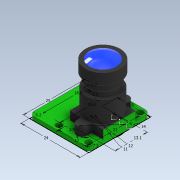
# Autodesk Inventor part: Arducam Camera
Saved by Autodesk Inventor 2020 (Build 240168000, 168)
## iProperties
Created: 2020-12-28
Part Number: Arducam Camera
Material: Generic
Document SubType Name: Modeling
Designer: DELL
Density: 1 g/cm^3
Appearance: Default
Author: DELL
Autodesk Inventor part; units mm, degrees
ref_plane "YZ Plane" through (0, 0, 0) normal (1, 0, 0) x (0, 1, 0)
ref_plane "XZ Plane" through (0, 0, 0) normal (0, 1, 0) x (-1, 0, 0)
ref_plane "XY Plane" through (0, 0, 0) normal (0, 0, 1) x (1, 0, 0)
sketch "Sketch1" plane through (0, 0, 0) normal (0, 1, 0) x (-1, 0, 0)
  line L0 (12, -12.5) -> (-12, -12.5)
  line L1 (-12, -12.5) -> (-12, 12.5)
  line L2 (-12, 12.5) -> (12, 12.5)
  line L3 (12, 12.5) -> (12, -12.5)
  line L4 (12, -12.5) -> (-12, 12.5) construction
  line L5 (-12, -12.5) -> (12, 12.5) construction
  circle A0 centre (2, 10.5) radius 1.25
  circle A1 centre (-10, 10.5) radius 1.25
  circle A2 centre (2, -10.5) radius 1.25
  circle A3 centre (-10, -10.5) radius 1.25
  line L6 (12, 0) -> (-12, 0) construction
  line L7 (10.1, -8.3) -> (11.8, -8.3)
  line L8 (11.8, -8.3) -> (11.8, 8.3)
  line L9 (11.8, 8.3) -> (10.1, 8.3)
  line L10 (10.1, 8.3) -> (10.1, -8.3)
  line L11 (10.1, -8.3) -> (11.8, 8.3) construction
  line L12 (11.8, -8.3) -> (10.1, 8.3) construction
  line L13 (6.6, -7.8) -> (10.1, -7.8)
  line L14 (10.1, -7.8) -> (10.1, 7.8)
  line L15 (10.1, 7.8) -> (6.6, 7.8)
  line L16 (6.6, 7.8) -> (6.6, -7.8)
  line L17 (6.6, -7.8) -> (10.1, 7.8) construction
  line L18 (10.1, -7.8) -> (6.6, 7.8) construction
  line L19 (1.5, -6.55) -> (-12, -6.55)
  line L20 (-12, -6.55) -> (-12, 6.55)
  line L21 (-12, 6.55) -> (1.5, 6.55)
  line L22 (1.5, 6.55) -> (1.5, -6.55)
  line L23 (1.5, -6.55) -> (-12, 6.55) construction
  line L24 (-12, -6.55) -> (1.5, 6.55) construction
  circle A4 centre (-5.25, 0) radius 6.75
  line L25 (-5.25, 6.55) -> (-5.25, -6.55) construction
  line L26 (-3.25, 8.55) -> (-3.25, -6.55)
  line L27 (-7.25, -8.55) -> (-7.25, 8.55)
  circle A5 centre (-5.25, 8.55) radius 2
  circle A6 centre (-5.25, -8.55) radius 2
  line L28 (-3.25, -8.55) -> (-3.25, -6.55)
  circle A7 centre (-5.25, 0) radius 6
  circle A8 centre (-5.25, 0) radius 5.5
  circle A9 centre (-5.25, 0) radius 7
  point P0 (0, 0)
  point P1 (10.95, 0)
  point P2 (8.35, 0)
  point P3 (-12, 1.854)
  point P4 (-12, -1.854)
  point P5 (-7.7193, -6.55)
  point P6 (-7.25, -6.7082)
  point P7 (-3.25, -6.7082)
  point P8 (-2.7807, -6.55)
  point P9 (-2.7807, 6.55)
  point P10 (-3.25, 6.7082)
  point P11 (-7.25, 6.7082)
  point P12 (-7.7193, 6.55)
  point P13 (12, -8.3)
  dimension "d0" = 25
  dimension "d1" = 24
  dimension "d2" = 2.5
  dimension "d3" = 21
  dimension "d4" = 12
  dimension "d5" = 2
  dimension "d6" = 16.6
  dimension "d7" = 1.7
  dimension "d8" = 15.6
  dimension "d9" = 3.5
  dimension "d10" = 13.5
  dimension "d11" = 13.1
  dimension "d12" = 4
  dimension "d13" = 4
  dimension "d14" = 11
  dimension "d15" = 12
  dimension "d16" = 14
  dimension "d35" = 0.2
  constraints: 58 end point, 12 midpoint, 9 centre point, 9 parallel, 6 point on line, 5 perpendicular, 4 coincident, 4 equal radius, 4 horizontal, 4 point on circle, 4 tangent, 3 horizontal alignment, 2 symmetric about line, 2 vertical alignment, 1 vertical, 3 other
  measures "d0" distance of L2.end L0.start
  measures "d1" distance of L1.end L2.end
  measures "d2" diameter of A0
  measures "d3" distance of A3.centre A1.centre
  measures "d4" distance of A1.centre A0.centre
  measures "d5" distance from line of L1 A1.centre
  measures "d6" distance between parallel lines of L7 L9
  measures "d7" distance of L7.start L7.end
  measures "d8" distance of L15.end L13.start
  measures "d9" distance of L13.start L13.end
  measures "d10" distance of L19.start L19.end
  measures "d11" distance of L21.end L19.start
  measures "d12" distance between parallel lines of L27 L26
  measures "d13" diameter of A5
  measures "d14" diameter of A8
  measures "d15" diameter of A7
  measures "d16" diameter of A9
  measures "d35" distance between parallel lines of L3 L8
extrude "Extrusion1" add sketch "Sketch1" along normal blind 1.6 contours L0 L1 L19 A9 L27 A6 L28 L22 L21 L26 A5 L2 L3 | L1 A9 L19 | L1 A4 L27 L19 A9 | L19 L27 A9 | L21 A9 L1 | L1 A9 L21 L27 A4 | A4 L27 A7 | L27 A4 L19 | L19 A4 A6 A9 L27 | A9 A6 L27 | A9 L27 L21 | L27 L21 A4 | A4 L21 L26 A7 L27 | L27 A7 L26 A4 L19 | L19 A6 A4 | A6 A9 | A6 A4 A9 | L27 A9 A5 A4 L21 | L27 A5 A9 | A4 A5 L21 | A7 L26 A8 L27 | L27 A8 A7 | L27 A8 L26 A7 | L19 A4 A6 | A6 A4 | A6 A9 L28 | A6 A4 L19 L28 A9 | A5 A9 | A9 A5 A4 | A5 A4 L21 | A5 A4 | A8 L26 L27 | L27 A8 | A7 L26 A8 | L26 A4 A7 | A4 L26 L19 | L28 L19 A9 | L26 A9 A5 | A9 L26 L21 A4 A5 | L21 L26 A4 | A8 L26 | L26 L21 A9 L22 A4 | A4 L22 A9 L19 L26 | A9 L22 L19 | A9 L21 L26 | L22 A9 | L21 L22 A9 | L10 L9 L8 L7 | L13 L16 L15 L10
extrude "Extrusion2" add sketch "Sketch1" along normal blind 3.5 from surface at 1.6 contours L1 A9 L19 | L1 A4 L27 L19 A9 | L19 L27 A9 | L21 A9 L1 | L1 A9 L21 L27 A4 | A4 L27 A7 | L27 A4 L19 | L19 A4 A6 A9 L27 | A9 A6 L27 | A9 L27 L21 | L27 L21 A4 | A4 L21 L26 A7 L27 | L27 A7 L26 A4 L19 | L19 A6 A4 | A6 A9 | A6 A4 A9 | L27 A9 A5 A4 L21 | L27 A5 A9 | A4 A5 L21 | A7 L26 A8 L27 | L27 A8 A7 | L27 A8 L26 A7 | L19 A4 A6 | A6 A4 | A6 A9 L28 | A6 A4 L19 L28 A9 | A5 A9 | A9 A5 A4 | A5 A4 L21 | A5 A4 | A8 L26 L27 | L27 A8 | A7 L26 A8 | L26 A4 A7 | A4 L26 L19 | L28 L19 A9 | L26 A9 A5 | A9 L26 L21 A4 A5 | L21 L26 A4 | A8 L26 | L26 L21 A9 L22 A4 | A4 L22 A9 L19 L26 | A9 L22 L19 | A9 L21 L26 | L21 L22 A9
extrude "Extrusion3" add sketch "Sketch1" along normal blind 8.5 from surface at 5.1 contours A4 L27 A7 | A4 L21 L26 A7 L27 | L27 A7 L26 A4 L19 | L19 A6 A4 | A4 A5 L21 | A7 L26 A8 L27 | L27 A8 A7 | L27 A8 L26 A7 | L19 A4 A6 | A6 A4 | A5 A4 L21 | A5 A4 | A8 L26 L27 | L27 A8 | A7 L26 A8 | L26 A4 A7 | A8 L26
extrude "Extrusion4" add sketch "Sketch1" along normal blind 2.4 from surface at 13.6 contours A8 L26 L27 | L27 A8 | A8 L26
extrude "Extrusion5" add sketch "Sketch1" along normal blind 2.8 from surface at 16 contours A7 L26 A8 L27 | L27 A8 A7 | L27 A8 L26 A7 | A8 L26 L27 | L27 A8 | A7 L26 A8 | A8 L26
extrude "Extrusion6" add sketch "Sketch1" along normal blind 4.5 from surface at 18.8 contours A9 L1 | L1 A4 L27 L19 A9 | L19 L27 A9 | L1 A9 L21 L27 A4 | A4 L27 A7 | L27 A4 L19 | L19 A4 A6 A9 L27 | A9 L27 L21 | L27 L21 A4 | A4 L21 L26 A7 L27 | L27 A7 L26 A4 L19 | L19 A6 A4 | A6 A4 A9 | L27 A9 A5 A4 L21 | A4 A5 L21 | A7 L26 A8 L27 | L27 A8 A7 | L27 A8 L26 A7 | L19 A4 A6 | A6 A4 | A6 A4 L19 L28 A9 | A9 A5 A4 | A5 A4 L21 | A5 A4 | A8 L26 L27 | L27 A8 | A7 L26 A8 | L26 A4 A7 | A4 L26 L19 | L28 L19 A9 | A9 L26 L21 A4 A5 | L21 L26 A4 | A8 L26 | L26 L21 A9 L22 A4 | A4 L22 A9 L19 L26 | A9 L21 L26 | L22 A9
extrude "Extrusion7" add sketch "Sketch1" against normal blind 2 contours L10 L9 L8 L7 | L13 L16 L15 L10
fillet "Fillet1" radius 2 4 edges at (-12, 0.8, -12.5) (-12, 0.8, 12.5) (12, 0.8, 12.5) (12, 0.8, -12.5)
sketch "Sketch2" plane through (0, 0, 0) normal (0, 0, 1) x (1, 0, 0)
  line L0 (-1.75, 23.3) -> (12.25, 23.3) projected
  line L1 (5.25, 23.3) -> (5.25, 0)
  line L2 (-10, 0) -> (10, 0) projected
  arc A0 (10.75, 23.3) -> (-0.25, 23.3) centre (5.25, 12.6346) ccw
  line L3 (10.75, 23.3) -> (-0.25, 23.3)
  line L4 (5.25, 23.3) -> (5.25, 24.6346)
  point P0 (0, 0)
  dimension "d32" = 1.5
  dimension "d33" = 12
  constraints: 6 end point, 3 point on circle, 3 point on line, 1 centre point, 1 collinear, 1 midpoint, 1 symmetric about line, 1 vertical
  measures "d32" distance of L0.end L3.start
  measures "d33" radius of A0
revolve "Revolution1" add sketch "Sketch2" angle 360 about axis through (5.25, 23.3, 0) along (0, 1, 0) picked at (8.3318, 23.5451) contours L4 A0 L0
body "Solid1"
